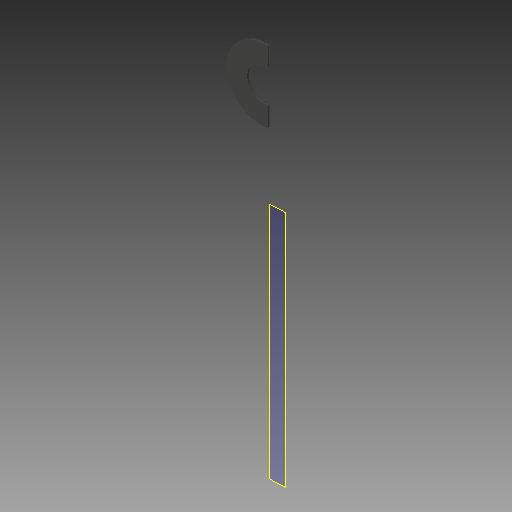
# Autodesk Inventor part: bue
Saved by Autodesk Inventor 2018 (Build 220112000, 112)
## iProperties
Created: 2020-08-13
Part Number: bue
Material: Steel
Document SubType Name: Sheet Metal
Designer: loppen
Density: 7.85 g/cm^3
Sheet Metal Rule: Default_mm
Appearance: Generic
Author: loppen
Autodesk Inventor part; units mm, degrees
ref_plane "YZ Plane" through (0, 0, 0) normal (1, 0, 0) x (0, 1, 0)
ref_plane "XZ Plane" through (0, 0, 0) normal (0, 1, 0) x (-1, 0, 0)
ref_plane "XY Plane" through (0, 0, 0) normal (0, 0, 1) x (1, 0, 0)
ref_plane "Work Plane1" through (-21.154, 0, -3.7385) normal (-0.039984, 0, -0.9992003) x (-0.9992003, 0, 0.039984)
sketch "Sketch1" plane through (-21.154, 0, -3.7385) normal (-0.039984, 0, -0.9992003) x (-0.9992003, 0, 0.039984)
  line L0 (1.0346, 490) -> (0.9998, 490)
  line L1 (0.9998, 0) -> (0.9998, 490)
  line L2 (1.0346, 0) -> (0.9998, 0)
  line L3 (1.0346, 0) -> (1.0346, 490)
  line L4 (0.9998, 540) -> (1.0346, 540)
  line L5 (1.0346, 540) -> (1.0346, 879.5354)
  line L6 (1.0346, 879.5354) -> (0.9998, 879.5354)
  line L7 (0.9998, 540) -> (0.9998, 879.5354)
  line L8 (1.0346, 540) -> (7.0346, 540)
  line L9 (0.9998, 490) -> (7.0346, 490)
  arc A0 (7.0346, 490) -> (7.0346, 540) centre (7.0346, 515) ccw
  line L10 (1.0346, 570) -> (7.0346, 570)
  arc A1 (7.0346, 460) -> (7.0346, 570) centre (7.0346, 515) ccw
  line L11 (7.0346, 460) -> (0.9998, 460)
  line L12 (1.0346, 570) -> (1.0346, 540)
  line L13 (0.9998, 490) -> (0.9998, 460)
  point P0 (-20.9876, 0)
  dimension "d0" = 30
  dimension "d1" = 6
  measures "d0" radial gap between concentric circles of A1 A0
  measures "d1" distance from line of L3 A0.centre
extrude "Plate1" add sketch "Sketch1" against normal blind 4 contours L3 L11 L1 L0 | L9 A0 L8 L5 L10 A1 L11 L3
equation "\"d2\" = Thickness"
equation "\"BendRadius\" = Thickness"
equation "\"BendReliefWidth\" = Thickness"
equation "\"BendReliefDepth\" = 0.5 * Thickness"
equation "\"CornerReliefSize\" = 4 * Thickness"
equation "\"MinimumRemnant\" = 2 * Thickness"
equation "\"TransitionRadius\" = BendRadius"
equation "\"JacobiRadiusSize\" = BendRadius"
equation "\"GapSize\" = Thickness"
equation "\"Thickness\" = 4"
body "Solid1"
